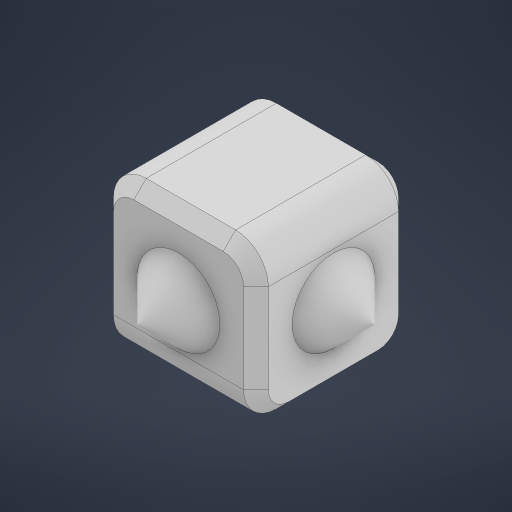
# Autodesk Inventor part: Universal_Joint
Saved by Autodesk Inventor 2024 (Build 280153000, 153)
## iProperties
Created: 2025-09-10
Part Number: Universal_Joint
Material: Generic
Document SubType Name: Modeling
Designer: kevin
Density: 1 g/cm^3
Appearance: Default
Author: kevin
Autodesk Inventor part; units mm, degrees
ref_plane "YZ Plane" through (0, 0, 0) normal (1, 0, 0) x (0, 1, 0)
ref_plane "XZ Plane" through (0, 0, 0) normal (0, 1, 0) x (-1, 0, 0)
ref_plane "XY Plane" through (0, 0, 0) normal (0, 0, 1) x (1, 0, 0)
sketch "Sketch1" plane through (0, 0, 0) normal (0, 1, 0) x (-1, 0, 0)
  line L0 (-7.5, 7.5) -> (7.5, 7.5)
  line L1 (7.5, 7.5) -> (7.5, -7.5)
  line L2 (7.5, -7.5) -> (-7.5, -7.5)
  line L3 (-7.5, -7.5) -> (-7.5, 7.5)
  line L4 (-7.5, 7.5) -> (7.5, -7.5) construction
  line L5 (7.5, 7.5) -> (-7.5, -7.5) construction
  point P0 (0, 0)
  dimension "d0" = 15
  dimension "d1" = 15
  constraints: 12 end point, 2 midpoint, 2 parallel, 1 horizontal, 1 perpendicular
  measures "d0" distance of L1.end L2.end
  measures "d1" distance of L0.end L1.end
extrude "Extrusion1" add sketch "Sketch1" along normal blind 15
sketch "Sketch2" plane through (-7.5, 0, 7.5) normal (0, 0, 1) x (1, 0, 0)
  line L0 (0, 0) -> (15, 0) projected
  line L1 (15, 0) -> (15, 15) projected
  line L2 (0, 15) -> (15, 15) projected
  line L3 (0, 0) -> (0, 15) projected
  line L4 (0, 15) -> (15, 0) construction
  circle A0 centre (7.5, 7.5) radius 4
  point P0 (7.5, 0)
  dimension "d4" = 8
  constraints: 2 end point, 1 centre point, 1 midpoint
  measures "d4" diameter of A0
sketch "Sketch3" plane through (0, 0, 0) normal (1, 0, 0) x (0, 1, 0)
  line L0 (0, 7.5) -> (0, -7.5) projected
  line L1 (0, -7.5) -> (15, -7.5) projected
  line L2 (15, 7.5) -> (15, -7.5) projected
  line L3 (0, 7.5) -> (15, 7.5) projected
  line L4 (7.5, 7.5) -> (7.5, 11.5)
  line L5 (7.5, 11.5) -> (11.5053, 7.5)
  point P0 (0, 0)
  dimension "d5" = 4
  constraints: 4 end point, 1 midpoint, 1 point on line, 1 vertical
  measures "d5" distance of L4.start L4.end
revolve "Revolution1" add sketch "Sketch3" angle 360 about axis through (0, 7.5, 7.5) along (0, 0, 1) contours L4 L5 L3
mirror "Mirror1" about plane through (0, 0, 0) normal (0, 0, 1) of "Revolution1"
fillet "Fillet1" radius 3.175 4 edges at (0, 0, 7.5) (7.5, 15, 0) (0, 0, -7.5) (-7.5, 15, 0)
chamfer "Chamfer1" distance 1.2 angle 45 16 edges at (-7.5, 7.5, 7.5) (-6.5701, 14.0701, 7.5) (0, 15, 7.5) (6.5701, 14.0701, 7.5) (7.5, 7.5, 7.5) (7.5, 0.9299, 6.5701) (7.5, 0, 0) (7.5, 0.9299, -6.5701) (7.5, 7.5, -7.5) (6.5701, 14.0701, -7.5) (0, 15, -7.5) (-6.5701, 14.0701, -7.5) (-7.5, 7.5, -7.5) (-7.5, 0.9299, -6.5701) (-7.5, 0, 0) (-7.5, 0.9299, 6.5701)
sketch "Sketch4" plane through (0, 0, 0) normal (0, 0, 1) x (1, 0, 0)
  circle A0 centre (0, 7.5) radius 4.0053 projected
  line L0 (-7.5, 3.175) -> (-7.5, 11.825) projected
  line L1 (-7.5, 7.5) -> (-11.5, 7.5)
  line L2 (-7.5, 7.5) -> (-7.5, 11.5)
  line L3 (-7.5, 11.5) -> (-11.5, 7.5)
  point P0 (0, 0)
  dimension "d11" = 4
  dimension "d12" = 4
  constraints: 6 end point, 1 horizontal, 1 midpoint, 1 point on line
  measures "d11" distance of L1.start L1.end
  measures "d12" distance of L1.start L2.end
revolve "Revolution2" add sketch "Sketch4" angle 360 about axis through (-7.5, 7.5, 0) along (-1, 0, 0) contours L1 L3 L0
mirror "Mirror2" about plane through (0, 0, 0) normal (1, 0, 0) of "Revolution2"
body "Solid1"
